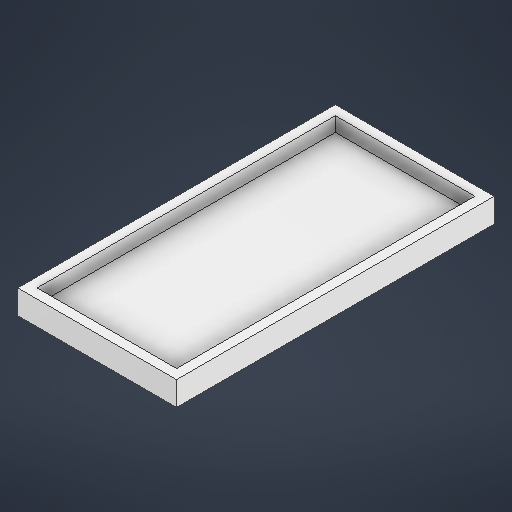
# Autodesk Inventor part: Deksel sensor
Saved by Autodesk Inventor 2026.2 (Build 302298000, 298)
## iProperties
Created: 2026-05-05
Part Number: Deksel sensor
Material: ABS Plastic
Document SubType Name: Modeling
Designer: Gameb
Density: 1.06 g/cm^3
Appearance: Smooth - White
Author: Gameb
Autodesk Inventor part; units mm, degrees
ref_plane "YZ Plane" through (0, 0, 0) normal (1, 0, 0) x (0, 1, 0)
ref_plane "XZ Plane" through (0, 0, 0) normal (0, 1, 0) x (-1, 0, 0)
ref_plane "XY Plane" through (0, 0, 0) normal (0, 0, 1) x (1, 0, 0)
sketch "Sketch1" plane through (0, 0, 0) normal (0, 1, 0) x (-1, 0, 0)
  line L0 (29, 62) -> (-29, 62)
  line L1 (-29, 62) -> (-29, -62)
  line L2 (-29, -62) -> (29, -62)
  line L3 (29, -62) -> (29, 62)
  line L4 (29, 62) -> (33, 62)
  line L5 (33, 62) -> (33, 66)
  line L6 (33, 66) -> (29, 66)
  line L7 (29, 66) -> (29, 62)
  line L8 (29, -62) -> (33, -62)
  line L9 (33, -62) -> (33, -66)
  line L10 (33, -66) -> (29, -66)
  line L11 (29, -66) -> (29, -62)
  line L12 (-29, -62) -> (-29, -66)
  line L13 (-29, -66) -> (-33, -66)
  line L14 (-33, -66) -> (-33, -62)
  line L15 (-33, -62) -> (-29, -62)
  line L16 (-29, 62) -> (-33, 62)
  line L17 (-33, 62) -> (-33, 66)
  line L18 (-33, 66) -> (-29, 66)
  line L19 (-29, 66) -> (-29, 62)
  line L20 (29, 66) -> (-29, 66)
  line L21 (-33, 62) -> (-33, -62)
  line L22 (-29, -66) -> (29, -66)
  line L23 (33, -62) -> (33, 62)
  line L24 (-33, 66) -> (-32.8039, 66)
  point P0 (0, 0)
  dimension "d2" = 58
  dimension "d3" = 124
  dimension "d5" = 4
  dimension "d6" = 4
  dimension "d7" = 4
  dimension "d8" = 4
  dimension "d9" = 4
  dimension "d10" = 4
  dimension "d11" = 4
  constraints: 50 end point, 10 point on line, 7 perpendicular, 4 horizontal, 4 parallel, 1 collinear, 1 vertical
  measures "d2" distance of L2.end L1.end
  measures "d3" distance of L1.end L0.end
  measures "d5" distance of L0.start L4.end
  measures "d6" distance of L4.end L5.end
  measures "d7" distance of L2.end L8.end
  measures "d8" distance of L8.end L9.end
  measures "d9" distance of L1.end L12.end
  measures "d10" distance of L12.end L13.end
  measures "d11" distance of L0.end L16.end
extrude "Extrusion1" add sketch "Sketch1" against normal blind 4
extrude "Extrusion2" add sketch "Sketch1" along normal blind 6 contours L4 L23 L8 L3 | L7 L6 L5 L4 | L0 L19 L20 L7 | L1 L15 L21 L16 | L16 L17 L18 L19 | L11 L22 L12 L2 | L8 L9 L10 L11 | L12 L13 L14 L15
body "Solid1"
